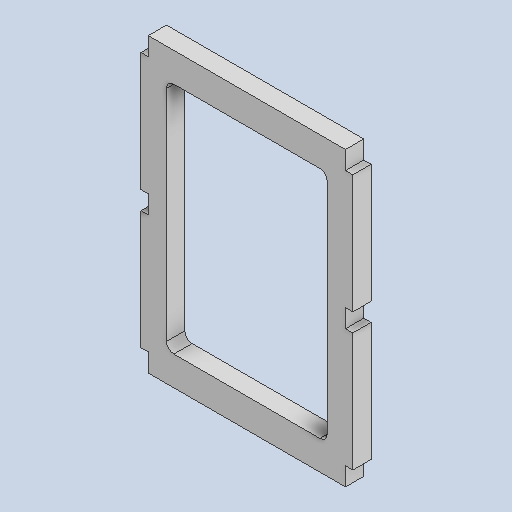
# Autodesk Inventor part: foot_connect
Saved by Autodesk Inventor 2022 (Build 260153000, 153)
## iProperties
Created: 2022-10-18
Part Number: foot_connect
Material: 一般
Document SubType Name: Modeling
Designer: haya
Density: 1 g/cm^3
Appearance: 既定
Author: haya
Autodesk Inventor part; units mm, degrees
ref_plane "YZ Plane" through (0, 0, 0) normal (1, 0, 0) x (0, 1, 0)
ref_plane "XZ Plane" through (0, 0, 0) normal (0, 1, 0) x (-1, 0, 0)
ref_plane "XY Plane" through (0, 0, 0) normal (0, 0, 1) x (1, 0, 0)
sketch "スケッチ1" plane through (0, 0, 0) normal (0, 0, 1) x (1, 0, 0)
  line L0 (0, 0) -> (54, 0)
  line L1 (54, 0) -> (54, 80)
  line L2 (54, 80) -> (0, 80)
  line L3 (0, 80) -> (0, 0)
  dimension "d0" = 54
  dimension "d1" = 80
  constraints: 8 end point, 2 parallel, 1 horizontal, 1 perpendicular
  measures "d0" distance of L0.start L0.end
  measures "d1" distance of L2.end L0.start
extrude "押し出し1" add sketch "スケッチ1" along normal blind 5
sketch "スケッチ2" plane through (54, 0, 0) normal (1, 0, 0) x (0, 0, -1)
  line L0 (0, 0) -> (0, 80) projected
  line L1 (0, 80) -> (-5, 80) projected
  line L2 (-5, 0) -> (-5, 80) projected
  line L3 (0, 0) -> (-5, 0) projected
  line L4 (-5, 0) -> (-5, 80) projected
  line L5 (-5, 40) -> (0, 40) construction
  line L6 (0, 0) -> (0, 80) projected
  line L7 (-5, 75) -> (0, 75)
  line L8 (0, 75) -> (0, 42.5)
  line L9 (0, 42.5) -> (-5, 42.5)
  line L10 (-5, 42.5) -> (-5, 75)
  line L11 (-5, 5) -> (0, 5)
  line L12 (0, 5) -> (0, 37.5)
  line L13 (0, 37.5) -> (-5, 37.5)
  line L14 (-5, 37.5) -> (-5, 5)
  point P0 (0, 37.5)
  point P1 (-5, 37.5)
  point P2 (0, 5)
  point P3 (-5, 42.5)
  point P4 (0, 42.5)
  point P5 (0, 75)
  dimension "d4" = 5
  dimension "d5" = 5
  constraints: 18 end point, 4 symmetric about line, 2 midpoint, 2 parallel, 2 point on line, 1 horizontal, 1 perpendicular
  measures "d4" distance between parallel lines of L7 L1
  measures "d5" distance between parallel lines of L13 L9
extrude "押し出し2" add sketch "スケッチ2" along normal blind 2 contours L11 L2 L13 L0 | L9 L2 L7 L0
sketch "スケッチ3" plane through (0, 0, 0) normal (-1, 0, 0) x (0, 0, 1)
  line L0 (0, 42.5) -> (0, 75) projected
  line L1 (0, 75) -> (5, 75) projected
  line L2 (5, 75) -> (5, 42.5) projected
  line L3 (5, 42.5) -> (0, 42.5) projected
  line L4 (5, 37.5) -> (5, 5) projected
  line L5 (5, 5) -> (0, 5) projected
  line L6 (0, 5) -> (0, 37.5) projected
  line L7 (0, 37.5) -> (5, 37.5) projected
  point P0 (0, 0)
extrude "押し出し3" add sketch "スケッチ3" along normal blind 2
sketch "スケッチ4" plane through (0, 0, 5) normal (0, 0, 1) x (1, 0, 0)
  line L0 (54, 0) -> (54, 5) projected
  line L1 (54, 5) -> (56, 5) projected
  line L2 (56, 37.5) -> (56, 5) projected
  line L3 (54, 37.5) -> (56, 37.5) projected
  line L4 (54, 37.5) -> (54, 42.5) projected
  line L5 (54, 42.5) -> (56, 42.5) projected
  line L6 (56, 75) -> (56, 42.5) projected
  line L7 (54, 75) -> (56, 75) projected
  line L8 (54, 75) -> (54, 80) projected
  line L9 (54, 80) -> (0, 80) projected
  line L10 (0, 80) -> (0, 75) projected
  line L11 (0, 75) -> (-2, 75) projected
  line L12 (-2, 42.5) -> (-2, 75) projected
  line L13 (0, 42.5) -> (-2, 42.5) projected
  line L14 (0, 42.5) -> (0, 37.5) projected
  line L15 (0, 37.5) -> (-2, 37.5) projected
  line L16 (-2, 5) -> (-2, 37.5) projected
  line L17 (0, 5) -> (-2, 5) projected
  line L18 (0, 5) -> (0, 0) projected
  line L19 (0, 0) -> (54, 0) projected
  line L20 (54, 80) -> (0, 80) projected
  line L21 (27, 80) -> (27, 0) construction
  line L22 (0, 0) -> (54, 0) projected
  line L23 (5, 72) -> (49, 72)
  line L24 (49, 72) -> (49, 8)
  line L25 (49, 8) -> (5, 8)
  line L26 (5, 8) -> (5, 72)
  line L27 (0, 42.5) -> (0, 37.5) projected
  line L28 (0, 40) -> (54, 40) construction
  dimension "d10" = 8
  dimension "d11" = 5
  constraints: 12 end point, 4 midpoint, 2 parallel, 1 horizontal, 1 perpendicular, 2 other
  measures "d10" distance between parallel lines of L23 L9
  measures "d11" distance between parallel lines of L0 L24
extrude "押し出し4" cut sketch "スケッチ4" against normal through all contours L23 L24 L25 L26
fillet "フィレット1" radius 2 4 edges at (49, 72, 2.5) (5, 72, 2.5) (5, 8, 2.5) (49, 8, 2.5)
